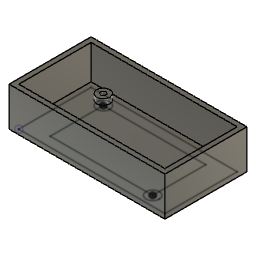
power-supply-housing (Autodesk Fusion 360 design; units mm, degrees)
Autodesk Fusion 360 part; units mm, degrees
note: some values were not read from the file. Set by a fixed rule: which sketch regions a step uses.
sketch "Sketch1" plane through (0, 0, 0) normal (0, 0, 1) x (1, 0, 0)
  line L0 (0, 0) -> (45, 0)
  line L1 (45, 0) -> (45, 22.25)
  line L2 (45, 22.25) -> (0, 22.25)
  line L3 (0, 22.25) -> (0, 0)
  line L4 (6.725, 2.955) -> (38.275, 2.955)
  line L5 (38.275, 2.955) -> (38.275, 19.295)
  line L6 (38.275, 19.295) -> (6.725, 19.295)
  line L7 (6.725, 19.295) -> (6.725, 2.955)
  circle A0 centre (6.725, 19.295) radius 0.8
  circle A1 centre (6.725, 19.295) radius 2
  circle A2 centre (38.275, 2.955) radius 0.8
  circle A3 centre (38.275, 2.955) radius 2
  dimension "d3" = 45
  dimension "d4" = 22.25
  dimension "d30" = 16.34
  dimension "d31" = 2.955
  dimension "d33" = 1.6
  dimension "d34" = 4
  dimension "d35" = 1.6
  dimension "d36" = 4
  dimension "d37" = 31.55
  dimension "d38" = 6.725
  constraint horizontal L0
  constraint vertical L1
  constraint horizontal L2
  constraint vertical L3
  constraint coincident L0.start L3.end
  constraint horizontal L4
  constraint vertical L5
  constraint horizontal L6
  constraint vertical L7
  constraint coincident L6.end L7.start
  constraint concentric A0 A1
  constraint coincident L4.end L5.start
  constraint concentric A2 A3
  measures "d3" distance of L0.start L0.end
  measures "d4" distance of L0.start L2.end
  measures "d30" distance of L4 L6
  measures "d31" distance of L0 L4
  measures "d33" diameter of A0
  measures "d34" diameter of A1
  measures "d35" diameter of A2
  measures "d36" diameter of A3
  measures "d37" distance of L5 L7
  measures "d38" distance of L3 L7
extrude "Extrude1" add sketch "Sketch1" along normal blind 1.5 contours L0 L1 L2 L3 | L4 L5 L6 L7 A1 A3 | L4 L5 A2 A3 | L4 L5 A2 A3 | L6 L7 A0 A1 | L6 L7 A0 A1 | L4 L5 A2 | L4 L5 A2 | L6 L7 A0 | L6 L7 A0 makes body 1
extrude "Extrude4" add sketch "Sketch1" along normal blind 12 thin wall 1.5 on the left open curves L0 L1 L2 L3 bodies 1
extrude "Extrude5" add sketch "Sketch1" along normal blind 1.75 separate body contours L4 L5 A2 A3 | L4 L5 A2 A3 makes body 2
extrude "Extrude6" add sketch "Sketch1" along normal blind 1.75 separate body contours L6 L7 A0 A1 | L6 L7 A0 A1 makes body 3
extrude "Extrude7" add sketch "Sketch1" along normal blind 1.5 separate body contours L0 L1 L2 L3 | L4 L5 L6 L7 A1 A3 | L4 L5 A2 A3 | L4 L5 A2 A3 | L6 L7 A0 A1 | L6 L7 A0 A1 | L4 L5 A2 | L4 L5 A2 | L6 L7 A0 | L6 L7 A0 makes body 4
move_body "Move3" bodies 2 to x (1, 0, 0) y (0, 1, 0) z (0, 0, 1) at (0, 0, 1.5)
move_body "Move4" bodies 3 to x (1, 0, 0) y (0, 1, 0) z (0, 0, 1) at (0, 0, 1.5)
